rod_label_clip (Autodesk Fusion 360 design; units mm, degrees)
part number: 2026-09-05-07-00-16-324
Autodesk Fusion 360 part; units mm, degrees
sketch "Ring" plane through (0, 0, 0) normal (0, 1, 0) x (1, 0, 0)
  circle A0 centre (0, 0) radius 17.05
  circle A1 centre (0, 0) radius 19.45
  dimension "d155" = 34.1
  dimension "d156" = 38.9
  constraint coincident A0.centre A1.centre
  constraint concentric A0 A1
  measures "d155" diameter of A0
  measures "d156" diameter of A1
extrude "Ring (1)" add sketch "Ring" along normal mid plane 9
sketch "Mouth" plane through (0, 0, 0) normal (0, 1, 0) x (1, 0, 0)
  line L0 (0, 0) -> (42.3486, -24.45)
  line L1 (42.3486, -24.45) -> (0, -48.9)
  line L2 (0, -48.9) -> (-42.3486, -24.45)
  line L3 (-42.3486, -24.45) -> (0, 0)
  line L4 (0, 0) -> (0, -48.9) construction
  dimension "d159" = 48.9
  dimension "d160" = 48.9
  dimension "d161" = 48.9
  dimension "d162" = 60
  dimension "d163" = 60
  constraint coincident L0.start L3.end
  constraint vertical L4
  constraint coincident L1.end L2.start
  measures "d159" distance of L0.start L0.end
  measures "d160" distance of L0.start L2.end
  measures "d161" distance of L0.start L1.end
  measures "d162" angle of L0 L4
  measures "d163" angle of L3 L4
extrude "Mouth (1)" cut sketch "Mouth" along normal mid plane 19
sketch "Stem" plane through (0, 0, 0) normal (0, 1, 0) x (1, 0, 0)
  line L0 (12.6501, 13.209) -> (20.8135, 22.9377)
  line L1 (20.8135, 22.9377) -> (18.975, 24.4804)
  line L2 (18.975, 24.4804) -> (10.8116, 14.7517)
  line L3 (10.8116, 14.7517) -> (12.6501, 13.209)
  dimension "d166" = 12.6501
  dimension "d167" = 13.209
  dimension "d168" = 20.8135
  dimension "d169" = 22.9377
  dimension "d170" = 18.975
  dimension "d171" = 24.4804
  dimension "d172" = 10.8116
  dimension "d173" = 14.7517
  measures "d166" horizontal distance of origin L0.start
  measures "d167" vertical distance of origin L0.start
  measures "d168" horizontal distance of origin L0.end
  measures "d169" vertical distance of origin L0.end
  measures "d170" horizontal distance of origin L1.end
  measures "d171" vertical distance of origin L1.end
  measures "d172" horizontal distance of origin L2.end
  measures "d173" vertical distance of origin L2.end
extrude "Stem (1)" add sketch "Stem" along normal mid plane 9
sketch "Label face" plane through (0, 0, 0) normal (0, 1, 0) x (1, 0, 0)
  line L0 (20.8135, 22.9377) -> (39.4544, 45.153)
  line L1 (39.4544, 45.153) -> (37.6159, 46.6957)
  line L2 (37.6159, 46.6957) -> (18.975, 24.4804)
  line L3 (18.975, 24.4804) -> (20.8135, 22.9377)
  dimension "d176" = 20.8135
  dimension "d177" = 22.9377
  dimension "d178" = 39.4544
  dimension "d179" = 45.153
  dimension "d180" = 37.6159
  dimension "d181" = 46.6957
  dimension "d182" = 18.975
  dimension "d183" = 24.4804
  measures "d176" horizontal distance of origin L0.start
  measures "d177" vertical distance of origin L0.start
  measures "d178" horizontal distance of origin L0.end
  measures "d179" vertical distance of origin L0.end
  measures "d180" horizontal distance of origin L1.end
  measures "d181" vertical distance of origin L1.end
  measures "d182" horizontal distance of origin L2.end
  measures "d183" vertical distance of origin L2.end
extrude "Label face (1)" add sketch "Label face" along normal mid plane 58
equation "clipWidth = 9.0 mm" comment "ring and stem width along the rod"
equation "faceWidth = 58.0 mm" comment "label face width along the rod"
equation "rodOuterDiameter = 33.4 mm" comment "rod the clip snaps onto"
equation "clipClearance = 0.7 mm" comment "diametral, so the clip slides"
equation "clipWall = 2.4 mm" comment "ring wall thickness"
equation "mouthHalfAngleDeg = 60.0 deg" comment "half the mouth opening"
equation "paddleThickness = 2.4 mm" comment "stem and label face thickness"
equation "stemEndRadius = ( rodOuterDiameter + clipClearance + 2 * clipWall ) / 2 + stemLength" comment "derived: stem ends, label face begins"
equation "faceEndRadius = stemEndRadius + faceHeight" comment "derived: outer edge of the label face"
equation "paddleAngleDeg = 50.0 deg" comment "paddle drop below horizontal"
equation "stemStartRadius = ( rodOuterDiameter + clipClearance ) / 2 + clipWall / 2" comment "derived: stem starts mid ring wall"
equation "stemLength = 11.5 mm" comment "stem reach beyond the ring outer wall"
equation "faceHeight = 29.0 mm" comment "label face, from stem end outward"
equation "d155 = rodOuterDiameter + clipClearance"
equation "d156 = rodOuterDiameter + clipClearance + 2 * clipWall"
equation "d157 = clipWidth"
equation "d159 = ( ( rodOuterDiameter + clipClearance + 2 * clipWall ) / 2 + 5 mm ) / cos(mouthHalfAngleDeg)"
equation "d160 = ( ( rodOuterDiameter + clipClearance + 2 * clipWall ) / 2 + 5 mm ) / cos(mouthHalfAngleDeg)"
equation "d161 = ( ( rodOuterDiameter + clipClearance + 2 * clipWall ) / 2 + 5 mm ) / cos(mouthHalfAngleDeg)"
equation "d162 = mouthHalfAngleDeg"
equation "d163 = mouthHalfAngleDeg"
equation "d164 = clipWidth + 10 mm"
equation "d166 = stemStartRadius * cos(paddleAngleDeg) + paddleThickness / 2 * sin(paddleAngleDeg)"
equation "d167 = stemStartRadius * sin(paddleAngleDeg) - paddleThickness / 2 * cos(paddleAngleDeg)"
equation "d168 = stemEndRadius * cos(paddleAngleDeg) + paddleThickness / 2 * sin(paddleAngleDeg)"
equation "d169 = stemEndRadius * sin(paddleAngleDeg) - paddleThickness / 2 * cos(paddleAngleDeg)"
equation "d170 = stemEndRadius * cos(paddleAngleDeg) - paddleThickness / 2 * sin(paddleAngleDeg)"
equation "d171 = stemEndRadius * sin(paddleAngleDeg) + paddleThickness / 2 * cos(paddleAngleDeg)"
equation "d172 = stemStartRadius * cos(paddleAngleDeg) - paddleThickness / 2 * sin(paddleAngleDeg)"
equation "d173 = stemStartRadius * sin(paddleAngleDeg) + paddleThickness / 2 * cos(paddleAngleDeg)"
equation "d174 = clipWidth"
equation "d176 = stemEndRadius * cos(paddleAngleDeg) + paddleThickness / 2 * sin(paddleAngleDeg)"
equation "d177 = stemEndRadius * sin(paddleAngleDeg) - paddleThickness / 2 * cos(paddleAngleDeg)"
equation "d178 = faceEndRadius * cos(paddleAngleDeg) + paddleThickness / 2 * sin(paddleAngleDeg)"
equation "d179 = faceEndRadius * sin(paddleAngleDeg) - paddleThickness / 2 * cos(paddleAngleDeg)"
equation "d180 = faceEndRadius * cos(paddleAngleDeg) - paddleThickness / 2 * sin(paddleAngleDeg)"
equation "d181 = faceEndRadius * sin(paddleAngleDeg) + paddleThickness / 2 * cos(paddleAngleDeg)"
equation "d182 = stemEndRadius * cos(paddleAngleDeg) - paddleThickness / 2 * sin(paddleAngleDeg)"
equation "d183 = stemEndRadius * sin(paddleAngleDeg) + paddleThickness / 2 * cos(paddleAngleDeg)"
equation "d184 = faceWidth"
named bodies: "rod_label_clip"
